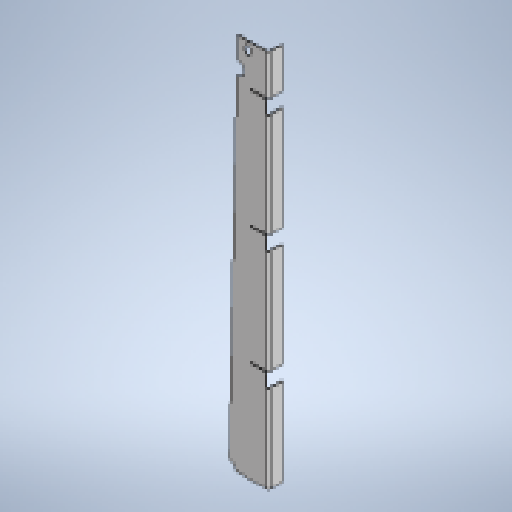
# Autodesk Inventor part: GBK 0201 second rib
Saved by Autodesk Inventor 2026.2 (Build 302298010, 298A)
## iProperties
Created: 2026-04-17
Part Number: GBK 0201 second rib
Material: Steel
Document SubType Name: Sheet Metal
Designer: pokla
Mass: 9637.89 g
Surface Area: 6317.93 cm^2
Volume: 1227.76 cm^3
Density: 7.85 g/cm^3
Sheet Metal Rule: Default
Appearance: Default
Flat Pattern Width: 21.9431 cm
Flat Pattern Length: 160.35 cm
Flat Pattern Area: 3518.59 cm^2
Sheet Metal Width: 219,431 mm
Sheet Metal Length: 1603,505 mm
Sheet Metal Area: 351859,104 mm^2
Author: admin
Autodesk Inventor part; units mm, degrees
ref_plane "YZ Plane" through (0, 0, 0) normal (1, 0, 0) x (0, 1, 0)
ref_plane "XZ Plane" through (0, 0, 0) normal (0, 1, 0) x (-1, 0, 0)
ref_plane "XY Plane" through (0, 0, 0) normal (0, 0, 1) x (1, 0, 0)
sketch "Sketch1" plane through (0, 0, 0) normal (0, 0, 1) x (1, 0, 0)
  line L0 (0, 0) -> (0, 1479.6195)
  line L1 (0, 1479.6195) -> (-162.4399, 1479.6195)
  line L2 (-162.4399, 1479.6195) -> (-196, 0)
  line L3 (-196, 0) -> (0, 0)
  line L4 (0, 410) -> (-5, 410)
  line L5 (-5, 410) -> (-5, 348.5)
  line L6 (-5, 348.5) -> (0, 348.5)
  line L7 (0, 348.5) -> (0, 410)
  line L8 (-5, 410) -> (-70, 410)
  line L9 (-70, 410) -> (-70, 405)
  line L10 (-70, 405) -> (-5, 405)
  line L11 (-5, 405) -> (-5, 410)
  line L12 (-70, 410) -> (-186.7006, 410) construction
  line L13 (0, 4408.8661) -> (0, 1479.6195)
  line L14 (-162.4399, 1479.6195) -> (-128.8798, 2959.2389)
  line L15 (0, 4408.8661) -> (-96, 4408.8661)
  line L16 (-128.8798, 2959.2389) -> (0, 2959.2389)
  line L17 (-128.8798, 2959.2389) -> (-96, 4408.8661)
  line L18 (-5, 848.5) -> (0, 848.5)
  line L19 (-70, 905) -> (-5, 905)
  line L20 (-5, 910) -> (-70, 910)
  line L21 (-70, 910) -> (-70, 905)
  line L22 (-5, 905) -> (-5, 910)
  line L23 (-5, 910) -> (-5, 848.5)
  line L24 (0, 848.5) -> (0, 910)
  line L25 (0, 910) -> (-5, 910)
  line L26 (-5, 1348.5) -> (0, 1348.5)
  line L27 (-70, 1405) -> (-5, 1405)
  line L28 (-5, 1410) -> (-70, 1410)
  line L29 (-70, 1410) -> (-70, 1405)
  line L30 (-5, 1405) -> (-5, 1410)
  line L31 (-5, 1410) -> (-5, 1348.5)
  line L32 (0, 1348.5) -> (0, 1410)
  line L33 (0, 1410) -> (-5, 1410)
  line L34 (-5, 1848.5) -> (0, 1848.5)
  line L35 (-70, 1905) -> (-5, 1905)
  line L36 (-5, 1910) -> (-70, 1910)
  line L37 (-70, 1910) -> (-70, 1905)
  line L38 (-5, 1905) -> (-5, 1910)
  line L39 (-5, 1910) -> (-5, 1848.5)
  line L40 (0, 1848.5) -> (0, 1910)
  line L41 (0, 1910) -> (-5, 1910)
  line L42 (-5, 2348.5) -> (0, 2348.5)
  line L43 (-70, 2405) -> (-5, 2405)
  line L44 (-5, 2410) -> (-70, 2410)
  line L45 (-70, 2410) -> (-70, 2405)
  line L46 (-5, 2405) -> (-5, 2410)
  line L47 (-5, 2410) -> (-5, 2348.5)
  line L48 (0, 2348.5) -> (0, 2410)
  line L49 (0, 2410) -> (-5, 2410)
  line L50 (-5, 2848.5) -> (0, 2848.5)
  line L51 (-70, 2905) -> (-5, 2905)
  line L52 (-5, 2910) -> (-70, 2910)
  line L53 (-70, 2910) -> (-70, 2905)
  line L54 (-5, 2905) -> (-5, 2910)
  line L55 (-5, 2910) -> (-5, 2848.5)
  line L56 (0, 2848.5) -> (0, 2910)
  line L57 (0, 2910) -> (-5, 2910)
  line L58 (-96, 4408.8661) -> (-95.3197, 4438.8584) construction
  line L59 (0, 1629.6195) -> (-159.0377, 1629.6195)
  line L60 (-126.158, 3079.2389) -> (0, 3079.2389)
  line L61 (-5, 3348.5) -> (0, 3348.5)
  line L62 (-70, 3405) -> (-5, 3405)
  line L63 (-5, 3410) -> (-70, 3410)
  line L64 (-70, 3410) -> (-70, 3405)
  line L65 (-5, 3405) -> (-5, 3410)
  line L66 (-5, 3410) -> (-5, 3348.5)
  line L67 (0, 3348.5) -> (0, 3410)
  line L68 (0, 3410) -> (-5, 3410)
  line L69 (-5, 3848.5) -> (0, 3848.5)
  line L70 (-70, 3905) -> (-5, 3905)
  line L71 (-5, 3910) -> (-70, 3910)
  line L72 (-70, 3910) -> (-70, 3905)
  line L73 (-5, 3905) -> (-5, 3910)
  line L74 (-5, 3910) -> (-5, 3848.5)
  line L75 (0, 3848.5) -> (0, 3910)
  line L76 (0, 3910) -> (-5, 3910)
  arc A0 (-136, 0) -> (-194.6395, 59.9846) centre (-196, 0) ccw
  arc A1 (-163.1202, 1449.6272) -> (-161.7596, 1509.6117) centre (-162.4399, 1479.6195) ccw
  arc A2 (-129.5601, 2929.2466) -> (-128.1995, 2989.2312) centre (-128.8798, 2959.2389) ccw
  line L77 (0, 910) -> (-70, 910)
  line L78 (-70, 910) -> (-175.3598, 910) construction
  line L79 (-70, 1410) -> (-164.019, 1410) construction
  line L80 (-70, 1910) -> (-152.6782, 1910) construction
  line L81 (-70, 2410) -> (-141.3374, 2410) construction
  line L82 (-70, 2910) -> (-129.9966, 2910) construction
  line L83 (-70, 3410) -> (-118.6558, 3410) construction
  line L84 (-70, 3910) -> (-107.3151, 3910) construction
  line L85 (-83.8875, 3050.2389) -> (-83.8875, 3040.2389) construction
  line L86 (-97.8875, 3050.2389) -> (-97.8875, 3040.2389)
  line L87 (-69.8875, 3040.2389) -> (-69.8875, 3050.2389)
  arc A3 (-69.8875, 3050.2389) -> (-97.8875, 3050.2389) centre (-83.8875, 3050.2389) ccw
  arc A4 (-97.8875, 3040.2389) -> (-69.8875, 3040.2389) centre (-83.8875, 3040.2389) ccw
  point P0 (-132.4399, 1479.6195)
  point P1 (-83.8875, 3045.2389)
  point P2 (-98.8875, 2958.5586)
  point P3 (-83.8875, 3026.2389)
  point P4 (-83.8875, 3064.2389)
  dimension "d25" = 410
  dimension "d32" = 1480
  dimension "d33" = 1480
  dimension "d34" = 1450
  dimension "d35" = 96
  dimension "d38" = 500
  dimension "d44" = 30
  dimension "d45" = 150
  dimension "d46" = 120
  dimension "d47" = 196
  dimension "d48" = 5
  dimension "d50" = 61.5
  dimension "d51" = 60
  dimension "d52" = 30
  dimension "d53" = 498.8661
  dimension "d54" = 30
  dimension "d56" = 186.7006
  dimension "d57" = 175.3598
  dimension "d58" = 164.019
  dimension "d59" = 152.6782
  dimension "d60" = 141.3374
  dimension "d61" = 129.9966
  dimension "d62" = 118.6559
  dimension "d63" = 107.3151
  dimension "d64" = 70
  dimension "d66" = 15
  dimension "d67" = 28
  dimension "d68" = 38
  dimension "d69" = 15
  measures "d25" distance between parallel lines of L3 L8
  measures "d32" distance of L2.end L1.end
  measures "d33" distance of L1.end L14.end
  measures "d34" distance of L14.end L15.end
  measures "d35" distance of L13.start L15.end
  measures "d38" distance of L6.start L18.start
  measures "d44" distance of L15.end L58.end
  measures "d45" distance between parallel lines of L1 L59
  measures "d46" distance between parallel lines of L16 L60
  measures "d47" distance of L2.end L0.start
  measures "d48" distance between parallel lines of L10 L8
  measures "d50" distance of L8.start L6.start
  measures "d51" radius of A0
  measures "d52" radius of A1
  measures "d53" distance from line of L71 L13.start
  measures "d54" radius of A2
  measures "d56" distance of L12.end L4.start
  measures "d57" distance of L78.end L24.end
  measures "d58" distance of L79.end L32.end
  measures "d59" distance of L80.end L40.end
  measures "d60" distance of L81.end L48.end
  measures "d61" distance of L82.end L56.end
  measures "d62" distance of L83.end L67.end
  measures "d63" distance of L84.end L75.end
  measures "d64" distance between parallel lines of L9 L0
  measures "d66" distance from line of point (-98.888, 2958.559) L85
  measures "d67" distance between parallel lines of L86 L87
  measures "d68" distance of point (-83.888, 3026.239) point (-83.888, 3064.239)
  measures "d69" distance from line of point (-83.888, 3064.239) L60
extrude "Plate1" add sketch "Sketch1" along normal blind 4 contours A1 L14 L59 L13 L1 | L14 A2 L16 L13 L57 L52 L53 L51 L55 L50 L49 L44 L45 L43 L47 L42 L41 L36 L37 L35 L39 L34 L59 | A2 L17 L60 L13 L16
sketch "Sketch2" plane through (4, 1479.6195, 4) normal (-1, 0, 0) x (0, -1, 0)
  line L0 (-368.8805, 0) -> (0, 0)
  line L1 (0, 0) -> (0, -60)
  line L2 (0, -60) -> (-368.8805, -60)
  line L3 (-368.8805, -60) -> (-368.8805, 0)
  constraints: 8 end point
edge flange "Flange1" height 60 angle 90 thickness 4 bend radius 4 thickness toward (-1, 0, 0) relief straight relief width 4 relief depth 2 corner gap 4 corner form 0 edges at (0, 1664.0597, 0) (0, 2129.25, 0) (0, 2629.25, 0) (0, 2994.6195, 0) wall of the first edge with corners at (4, 1848.5, 4) (4, 1479.6195, 4) (4, 1479.6195, -56) (4, 1848.5, -56)
bend "Bend1"
corner "Corner1"
chamfer "Corner Chamfer1" distance 10 angle 45 3 edges at (-5, 1905, 2) (-5, 2405, 2) (-5, 2905, 2)
equation "\"d5\" = Thickness"
equation "\"d7\" = BendReliefWidth"
equation "\"d8\" = BendReliefDepth"
equation "\"d9\" = MinimumRemnant"
equation "\"d10\" = TransitionRadius"
equation "\"d13\" = BendRadius"
equation "\"d14\" = CornerReliefSize"
equation "\"d15\" = GapSize"
equation "\"d16\" = JacobiRadiusSize"
equation "\"BendRadius\" = Thickness"
equation "\"BendReliefWidth\" = Thickness"
equation "\"BendReliefDepth\" = 0.5 * Thickness"
equation "\"CornerReliefSize\" = 4 * Thickness"
equation "\"MinimumRemnant\" = 2 * Thickness"
equation "\"TransitionRadius\" = BendRadius"
equation "\"JacobiRadiusSize\" = BendRadius"
equation "\"GapSize\" = Thickness"
equation "\"Thickness\" = 4"
body "Solid1"
